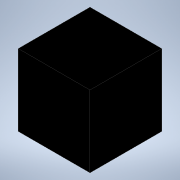
# Autodesk Inventor part: cube
Saved by Autodesk Inventor 2020 (Build 240168000, 168)
## iProperties
Created: 2020-12-12
Part Number: cube
Material: Типовые
Document SubType Name: Modeling
Designer: Trizo
Density: 1 g/cm^3
Appearance: По умолчанию
Author: Trizo
Autodesk Inventor part; units mm, degrees
ref_plane "YZ Plane" through (0, 0, 0) normal (1, 0, 0) x (0, 1, 0)
ref_plane "XZ Plane" through (0, 0, 0) normal (0, 1, 0) x (-1, 0, 0)
ref_plane "XY Plane" through (0, 0, 0) normal (0, 0, 1) x (1, 0, 0)
sketch "Эскиз1" plane through (0, 0, 0) normal (0, 0, 1) x (1, 0, 0)
  line L0 (250, -250) -> (-250, -250)
  line L1 (-250, -250) -> (-250, 250)
  line L2 (-250, 250) -> (250, 250)
  line L3 (250, 250) -> (250, -250)
  line L4 (250, -250) -> (-250, 250) construction
  line L5 (-250, -250) -> (250, 250) construction
  point P0 (0, 0)
  dimension "d0" = 500
  dimension "d1" = 500
  constraints: 12 end point, 2 midpoint, 2 parallel, 1 horizontal, 1 perpendicular
  measures "d0" distance of L1.end L2.end
  measures "d1" distance of L0.end L1.end
extrude "Выдавливание1" add sketch "Эскиз1" along normal mid plane 500
